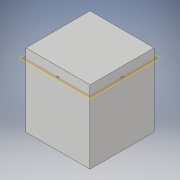
# Autodesk Inventor part: companion_cube
Saved by Autodesk Inventor 2017 (Build 210142000, 142)
## iProperties
Created: 2018-10-23
Part Number: companion_cube
Material: Generic
Document SubType Name: Modeling
Designer: jacob
Density: 1 g/cm^3
Appearance: Default
Author: jacob
Autodesk Inventor part; units mm, degrees
ref_plane "YZ Plane" through (0, 0, 0) normal (1, 0, 0) x (0, 1, 0)
ref_plane "XY Plane" through (0, 0, 0) normal (0, 0, 1) x (1, 0, 0)
sketch "Sketch1" plane through (0, 0, 0) normal (0, 1, 0) x (-1, 0, 0)
  line L0 (11.43, 11.43) -> (-11.43, 11.43)
  line L1 (-11.43, 11.43) -> (-11.43, -11.43)
  line L2 (-11.43, -11.43) -> (11.43, -11.43)
  line L3 (11.43, -11.43) -> (11.43, 11.43)
  line L4 (0.381, -11.43) -> (0.381, 11.43)
  line L5 (-0.381, -11.43) -> (-0.381, 11.43)
  line L6 (11.43, -0.381) -> (-11.43, -0.381)
  line L7 (11.43, 0.381) -> (-11.43, 0.381)
  circle A0 centre (0, 0) radius 5.08
  line L8 (12.446, -12.446) -> (-12.446, -12.446)
  line L9 (-12.446, -12.446) -> (-12.446, 12.446)
  line L10 (-12.446, 12.446) -> (12.446, 12.446)
  line L11 (12.446, 12.446) -> (12.446, -12.446)
  dimension "d0" = 22.86
  dimension "d1" = 22.86
  dimension "d2" = 11.43
  dimension "d3" = 11.43
  dimension "d7" = 0.381
  dimension "d8" = 0.762
  dimension "d12" = 0.381
  dimension "d13" = 0.381
  dimension "d14" = 0.762
  dimension "d21" = 10.16
  dimension "d28" = 1.016
  dimension "d29" = 1.016
  dimension "d30" = 1.016
  dimension "d31" = 1.016
  constraints: 24 end point, 8 point on line, 6 perpendicular, 4 parallel, 2 horizontal, 1 centre point, 1 coincident
  measures "d0" distance of L2.end L0.start
  measures "d1" distance of L1.end L2.end
  measures "d2" distance from line of point (0, 0) L0
  measures "d3" distance from line of point (0, 0) L3
  measures "d7" distance from line of point (0, 0) L4
  measures "d8" distance between parallel lines of L4 L5
  measures "d12" distance from line of point (0, 0) L6
  measures "d13" distance from line of point (0, 0) L7
  measures "d14" distance between parallel lines of L7 L6
  measures "d21" diameter of A0
  measures "d28" distance between parallel lines of L2 L8
  measures "d29" distance between parallel lines of L9 L1
  measures "d30" distance between parallel lines of L0 L10
  measures "d31" distance between parallel lines of L3 L11
extrude "Extrusion2" add sketch "Sketch1" against normal blind 22.86 contours L3 L7 A0 L4 L0 | L4 A0 L5 L0 | L3 L6 A0 L7 | L5 A0 L7 L1 L0 | A0 L7 L4 | L4 L7 L5 A0 | L3 L2 L4 A0 L6 | A0 L6 L4 L7 | L5 L7 A0 | L4 L6 L5 L7 | A0 L4 L6 | L7 A0 L6 L1 | L5 L6 A0 L7 | L4 A0 L5 L6 | L2 L5 A0 L4 | L6 A0 L5 L2 L1 | L5 A0 L6
extrude "Extrusion3" cut sketch "Sketch1" against normal blind 0.254 contours L4 A0 L5 L0 | L3 L6 A0 L7 | L4 L7 L5 A0 | A0 L6 L4 L7 | L4 L6 L5 L7 | L7 A0 L6 L1 | L5 L6 A0 L7 | L4 A0 L5 L6 | L2 L5 A0 L4
extrude "Extrusion4" add sketch "Sketch1" along normal blind 0.508 contours A0 L7 L4 | L4 L7 L5 A0 | A0 L6 L4 L7 | L5 L7 A0 | L4 L6 L5 L7 | A0 L4 L6 | L5 L6 A0 L7 | L4 A0 L5 L6 | L5 A0 L6
sketch "Sketch3" plane through (0, 0, 0) normal (0, 1, 0) x (-1, 0, 0)
  line L0 (11.43, -11.43) -> (11.43, -0.381) projected
  line L1 (-11.43, 11.43) -> (-11.43, 0.381) projected
  line L2 (11.43, -11.43) -> (-11.43, -11.43)
  line L3 (-11.43, -11.43) -> (-11.43, 11.43)
  line L4 (-11.43, 11.43) -> (11.43, 11.43)
  line L5 (11.43, 11.43) -> (11.43, -11.43)
  point P0 (0, 0)
  constraints: 8 end point, 2 parallel, 1 horizontal, 1 perpendicular
extrude "Extrusion5" add sketch "Sketch3" along normal blind 3.175
sketch "Sketch4" plane through (0, 0, 0) normal (0, 1, 0) x (-1, 0, 0)
  circle A0 centre (0, -0.381) radius 8.0989
  point P0 (0, 0)
  constraints: 1 centre point
body "Solid2"
